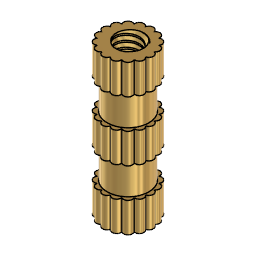
colour_detection_mechanism (Autodesk Fusion 360 archive; units mm, degrees)
design "M2 10 mm Threaded Brass Insert"
part number: 2026-06-20-09-24-02-047
Autodesk Fusion 360 part; units mm, degrees
sketch "Brass thread outline" plane through (0, 0, 0) normal (0, 0, 1) x (1, 0, 0)
  circle A0 centre (0, 0) radius 1.4
  dimension "d4" = 2.8
  constraint coincident A0.centre origin
  measures "d4" diameter of A0
extrude "Extrude1" add sketch "Brass thread outline" along normal blind 10
sketch "Ridges" plane through (0, 0, 10) normal (0, 0, 1) x (-1, 0, 0)
  circle A0 centre (0, 0) radius 1.4
  circle A1 centre (0, 0) radius 1.7
  circle A2 centre (-0.0001, -1.4) radius 0.3
  circle A3 centre (0.5357, -1.2935) radius 0.3
  circle A4 centre (0.9899, -0.99) radius 0.3
  circle A5 centre (1.2934, -0.5358) radius 0.3
  circle A6 centre (1.4, -0.0001) radius 0.3
  circle A7 centre (1.2935, 0.5357) radius 0.3
  circle A8 centre (0.99, 0.9899) radius 0.3
  circle A9 centre (0.5358, 1.2934) radius 0.3
  circle A10 centre (0.0001, 1.4) radius 0.3
  circle A11 centre (-0.5357, 1.2935) radius 0.3
  circle A12 centre (-0.9899, 0.99) radius 0.3
  circle A13 centre (-1.2934, 0.5358) radius 0.3
  circle A14 centre (-1.4, 0.0001) radius 0.3
  circle A15 centre (-1.2935, -0.5357) radius 0.3
  circle A16 centre (-0.99, -0.9899) radius 0.3
  circle A17 centre (-0.5358, -1.2934) radius 0.3
  dimension "d8" = 3.4
  dimension "d29" = 0.0001
  dimension "d31" = 360
  constraint coincident A0.centre A1.centre
  constraint coincident A0 A2.centre
  constraint tangent A1 A2
  measures "d8" diameter of A1
  measures "d29" horizontal distance of A0.centre A2.centre
extrude "Extrude2" add sketch "Ridges" against normal blind 2 contours A0 A5 A6 A7 | A0 A5 A6 A7 | A0 A6 A7 | A0 A6 A7 | A0 A5 A6 | A0 A5 A6 | A0 A6 A7 A8 | A0 A6 A7 A8 | A2 A3 A4 A5 A6 A7 A8 A9 A10 A11 A12 A13 A14 A15 A16 A17 | A0 A4 A5 A6 | A0 A4 A5 A6 | A0 A7 A8 | A0 A7 A8 | A0 A7 A8 A9 | A0 A4 A5 | A0 A4 A5 | A0 A3 A4 A5 | A0 A7 A8 A9 | A0 A8 A9 A10 | A0 A8 A9 | A0 A3 A4 A5 | A0 A2 A3 A4 | A0 A3 A4 | A0 A8 A9 | A0 A8 A9 A10 | A0 A9 A10 A11 | A0 A9 A10 | A0 A3 A4 | A0 A2 A3 A17 | A0 A2 A3 | A0 A2 A3 A4 | A0 A9 A10 | A0 A9 A10 A11 | A0 A10 A11 A12 | A0 A10 A11 | A0 A2 A3 | A0 A2 A17 | A0 A2 A16 A17 | A0 A2 A3 A17 | A0 A10 A11 | A0 A10 A11 A12 | A0 A11 A12 A13 | A0 A11 A12 | A0 A2 A16 A17 | A0 A2 A17 | A0 A15 A16 A17 | A0 A16 A17 | A0 A11 A12 | A0 A11 A12 A13 | A0 A16 A17 | A0 A15 A16 A17 | A0 A12 A13 | A0 A12 A13 | A0 A12 A13 A14 | A0 A14 A15 A16 | A0 A15 A16 | A0 A15 A16 | A0 A12 A13 A14 | A0 A14 A15 A16 | A0 A13 A14 | A0 A13 A14 | A0 A13 A14 A15 | A0 A13 A14 A15 | A0 A14 A15 | A0 A14 A15
pattern_linear "R-Pattern1" count 3 spacing 4 along (0, 0, -1) of "Extrude2"
sketch "Thread hole" plane through (0, 0, 10) normal (0, 0, 1) x (-1, 0, 0)
  circle A0 centre (0, 0) radius 1
  arc A1 (0.292, -1.4685) -> (0.8317, -1.2449) centre (0.5357, -1.2935) ccw
  arc A2 (0.8317, -1.2449) -> (1.2448, -0.8319) centre (0.9899, -0.99) ccw
  arc A3 (1.2448, -0.8319) -> (1.4684, -0.2922) centre (1.2934, -0.5358) ccw
  arc A4 (1.4684, -0.2922) -> (1.4685, 0.292) centre (1.4, -0.0001) ccw
  arc A5 (1.4685, 0.292) -> (1.2449, 0.8317) centre (1.2935, 0.5357) ccw
  arc A6 (1.2449, 0.8317) -> (0.8319, 1.2448) centre (0.99, 0.9899) ccw
  arc A7 (0.8319, 1.2448) -> (0.2922, 1.4684) centre (0.5358, 1.2934) ccw
  arc A8 (0.2922, 1.4684) -> (-0.292, 1.4685) centre (0.0001, 1.4) ccw
  arc A9 (-0.292, 1.4685) -> (-0.8317, 1.2449) centre (-0.5357, 1.2935) ccw
  arc A10 (-0.8317, 1.2449) -> (-1.2448, 0.8319) centre (-0.9899, 0.99) ccw
  arc A11 (-1.2448, 0.8319) -> (-1.4684, 0.2922) centre (-1.2934, 0.5358) ccw
  arc A12 (-1.4684, 0.2922) -> (-1.4685, -0.292) centre (-1.4, 0.0001) ccw
  arc A13 (-1.4685, -0.292) -> (-1.2449, -0.8317) centre (-1.2935, -0.5357) ccw
  arc A14 (-1.2449, -0.8317) -> (-0.8319, -1.2448) centre (-0.99, -0.9899) ccw
  arc A15 (-0.8319, -1.2448) -> (-0.2922, -1.4684) centre (-0.5358, -1.2934) ccw
  arc A16 (-0.2922, -1.4684) -> (0.292, -1.4685) centre (-0.0001, -1.4) ccw
  dimension "d11" = 2
  constraint coincident A0.centre origin
  measures "d11" diameter of A0
extrude "Extrude3" cut sketch "Thread hole" against normal blind 10 contours A0
thread "Thread1" "ISO Metric profile 2.0 M2x0.4 M2x0.4 6H" major diameter 2.074 minor diameter 1.623 pitch 0.4 angle 60 modelled right hand crest width 0.1065 on face at (-0.9988, 0.0498, 3.3333) crest through (-0.8115, 0, 9.9)
equation "outer_diameter = 2.8 mm" comment "The outer diameter of the non-ridged parts."
equation "hole_diameter = 2 mm" comment "The thread diameter of the brass insert. 2 mm for this M2 insert."
equation "height = 10 mm" comment "The height of the brass thread insert. 10 mm for this model."
equation "d4 = outer_diameter"
equation "d5 = height"
equation "ridge_diameter = 3.4 mm" comment "The outer diameter of the ridged parts."
equation "d8 = ridge_diameter"
equation "d9 = -ridge_height"
equation "d11 = hole_diameter"
equation "d12 = -height"
equation "number_of_ridges = 3" comment "The number of ridges to have along the outside."
equation "d23 = number_of_ridges"
equation "d25 = -ridge_pattern_length"
equation "ridge_pattern_length = height - ridge_height" comment "The distance to use for the rectangular pattern that repeats the ridges."
equation "ridge_height = 2 mm" comment "The height of the individual ridges."
named bodies: "M2 10 mm Threaded Brass Insert"

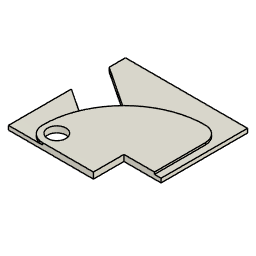
design "Colour Detection Mechanism Platform"
Autodesk Fusion 360 part; units mm, degrees
sketch "Colour Detection Mechanism Platform" plane through (0, 0, 0) normal (0, 0, 1) x (1, 0, 0)
  line L0 (0, 0) -> (120, 0)
  line L1 (120, 0) -> (120, 76)
  line L2 (120, 76) -> (0, 76)
  line L3 (0, 76) -> (0, 0)
  dimension "d169" = 120
  dimension "d170" = 76
  constraint horizontal L0
  constraint vertical L1
  constraint horizontal L2
  constraint vertical L3
  constraint coincident L0.start L3.end
  measures "d169" distance of L0.start L0.end
  measures "d170" distance of L0.start L2.end
extrude "Extrude42" add sketch "Colour Detection Mechanism Platform" along normal blind 4
sketch "Smartie Path" plane through (0, 0, 4) normal (0, 0, 1) x (-1, 0, 0)
  line L0 (0, -76) -> (0, 0)
  line L1 (0, 0) -> (-120, 0)
  line L2 (-120, 0) -> (-120, -76)
  line L3 (-120, -76) -> (0, -76)
  circle A0 centre (-98.5, 24) radius 80
  line L4 (-98.5, 24) -> (-113.5, 24)
  line L5 (-113.5, 24) -> (-113.5, -56)
  line L6 (-113.5, -56) -> (-98.5, -56)
  line L7 (-98.5, -56) -> (-98.5, 24)
  line L8 (-98.5, 24) -> (-18.5, 24)
  line L9 (-18.5, 24) -> (-18.5, 39)
  line L10 (-18.5, 39) -> (-98.5, 39)
  line L11 (-98.5, 39) -> (-98.5, 24)
  line L12 (-98.5, 24) -> (-113.5, 24)
  line L13 (-113.5, 24) -> (-113.5, 39)
  line L14 (-113.5, 39) -> (-98.5, 39)
  line L15 (-98.5, 39) -> (-98.5, 24)
  circle A1 centre (-32.5, 24) radius 9
  dimension "d173" = 160
  dimension "d174" = 24
  dimension "d175" = 21.5
  dimension "d176" = 15
  dimension "d177" = 15
  dimension "d178" = 80
  dimension "d179" = 80
  dimension "d184" = 18
  dimension "d185" = 14
  constraint horizontal L4
  constraint vertical L5
  constraint horizontal L6
  constraint vertical L7
  constraint coincident A0.centre L4.start
  constraint horizontal L8
  constraint vertical L9
  constraint horizontal L10
  constraint vertical L11
  constraint horizontal L12
  constraint vertical L13
  constraint horizontal L14
  constraint vertical L15
  constraint collinear L5 L13
  constraint collinear L10 L14
  constraint coincident L8 A1.centre
  measures "d173" diameter of A0
  measures "d174" distance of L1 A0.centre
  measures "d175" horizontal distance of L1.end A0.centre
  measures "d176" distance of L8.end L9.end
  measures "d177" distance of L5.end L6.end
  measures "d178" distance of L4.end L5.end
  measures "d179" distance of L9.end L10.end
  measures "d184" diameter of A1
  measures "d185" distance of L8.end A1.centre
extrude "Extrude43" add sketch "Smartie Path" along normal blind 2 contours L1 A0 L7 | L1 A0 L7 L8 A1 | L1 A0 L5 L7 | L1 L4 L5 L7 L12 | A0 L8 L10 L11 L15 A1 | L4 L11 L12 L13 L14 L15
fillet "Fillet2" radius 15 2 edges at (19.9188, -39, 5) (113.5, 54.5812, 5)
extrude "Extrude44" add 1 faces at (89.4665, -20.5529, 4) along direction (0, 0, -1) blind 4
sketch "Servo Hole" plane through (0, 0, 6) normal (0, 0, 1) x (-1, 0, 0)
  circle A0 centre (-32.5, 24) radius 9
  arc A1 (-113.5, -41) -> (-98.5, -56) centre (-98.5, -41) ccw
  arc A2 (-98.5, -56) -> (-18.5, 24) centre (-98.5, 24) ccw
  arc A3 (-18.5, 24) -> (-33.5, 39) centre (-33.5, 24) ccw
  line L0 (-33.5, 39) -> (-113.5, 39)
  line L1 (-113.5, 39) -> (-113.5, -41)
  line L2 (-113.5, 39) -> (-83.5, 39)
  line L3 (-83.5, 39) -> (-83.5, 9)
  line L4 (-83.5, 9) -> (-113.5, 9)
  line L5 (-113.5, 9) -> (-113.5, 39)
  dimension "d188" = 30
  dimension "d189" = 30
  constraint horizontal L2
  constraint vertical L3
  constraint horizontal L4
  constraint vertical L5
  constraint coincident L0.end L1.start
  measures "d188" distance of L3.end L4.end
  measures "d189" distance of L2.end L3.end
extrude "Extrude45" cut sketch "Servo Hole" against normal blind 6 contours L0 L1 L2 L3 L4 L5
sketch "Colour Sensor Holder Hole" plane through (0, 0, 4) normal (0, 0, 1) x (-1, 0, 0)
  line L0 (-120, 0) -> (-120, -76)
  line L1 (-120, -76) -> (0, -76)
  line L2 (0, -76) -> (0, 0)
  line L3 (-113.5, 0) -> (-120, 0)
  arc A0 (-98.5, -56) -> (-22.1849, 0) centre (-98.5, 24) ccw
  arc A1 (-113.5, -41) -> (-98.5, -56) centre (-98.5, -41) ccw
  line L4 (-113.5, -41) -> (-113.5, 0)
  line L5 (0, -59.401) -> (-38.732, -33.6675)
  line L6 (0, -23.4021) -> (-22.139, -8.693)
  line L7 (-38.732, -33.6675) -> (-22.139, -8.693)
  line L8 (0, -60.0013) -> (-39.4252, -33.8073)
  line L9 (-39.4252, -33.8073) -> (-22.2788, -7.9998)
  line L10 (-22.2788, -7.9998) -> (0, -22.8018)
  line L11 (0, 0) -> (-22.1849, 0)
  dimension "d249" = 56.4
  dimension "d250" = 59.401
  dimension "d254" = 56.4
  dimension "d255" = 8.693
  dimension "d256" = 22.139
  dimension "d257" = 23.4021
  dimension "d258" = 38.732
  dimension "d261" = 0.5
  dimension "d262" = 0.5
  dimension "d263" = 0.5
  constraint coincident L2 L5.start
  constraint coincident L2 L6.start
  constraint coincident L2 L8.start
  constraint coincident L2 L10.end
  constraint perpendicular L9 L10
  constraint parallel L5 L8
  constraint parallel L7 L9
  measures "d249" angle of L2 L5
  measures "d250" distance of L2.end L5.start
  measures "d254" angle of L2 L6
  measures "d255" distance of L3 L6.end
  measures "d256" horizontal distance of L2.end L6.end
  measures "d257" distance of L2.end L6.start
  measures "d258" horizontal distance of L5.start L5.end
  measures "d261" distance of L5 L8
  measures "d262" distance of L7 L9
extrude "Extrude58" cut sketch "Colour Sensor Holder Hole" against normal blind 4 contours L2 L5 L6 L7
extrude "Extrude59" cut sketch "Colour Sensor Holder Hole" against normal blind 4 contours L2 L5 L6 L7 L8 L9 L10
sketch "Platform Extension" plane through (0, 0, 4) normal (0, 0, 1) x (-1, 0, 0)
  line L0 (-22.2788, -7.9998) -> (0, -22.8018)
  line L1 (0, -22.8018) -> (0, 0)
  line L2 (0, 0) -> (-22.1849, 0)
  arc A0 (-98.5, -56) -> (-22.1849, 0) centre (-98.5, 24) ccw
  arc A1 (-113.5, -41) -> (-98.5, -56) centre (-98.5, -41) ccw
  line L3 (-113.5, -41) -> (-113.5, 0)
  line L4 (-120, 0) -> (-120, -76)
  line L5 (-120, -76) -> (0, -76)
  line L6 (0, -60.0013) -> (-39.4252, -33.8073)
  line L7 (-39.4252, -33.8073) -> (-22.2788, -7.9998)
  line L8 (-83.5, 9) -> (-113.5, 9)
  line L9 (-113.5, 9) -> (-113.5, -41)
  arc A2 (-113.5, -41) -> (-98.5, -56) centre (-98.5, -41) ccw
  arc A3 (-98.5, -56) -> (-18.5, 24) centre (-98.5, 24) ccw
  arc A4 (-18.5, 24) -> (-33.5, 39) centre (-33.5, 24) ccw
  line L10 (-33.5, 39) -> (-83.5, 39)
  line L11 (-83.5, 39) -> (-83.5, 9)
  circle A5 centre (-32.5, 24) radius 9
  line L12 (0, 0) -> (0, 39)
  line L13 (0, 39) -> (-33.5, 39)
  line L14 (-113.5, 0) -> (-120, 0)
  line L15 (0, -76) -> (0, -60.0013)
  line L16 (-113.5, 0) -> (-120, 0)
  line L17 (-120, 0) -> (-120, 9)
  line L18 (-120, 9) -> (-113.5, 9)
  line L19 (-113.5, 9) -> (-113.5, 0)
  constraint coincident L1.end L2.start
  constraint coincident A4.end L10.start
  constraint perpendicular L2 L12
  constraint perpendicular L12 L13
  constraint horizontal L16
  constraint vertical L17
  constraint horizontal L18
  constraint vertical L19
  constraint coincident L3.end L14.start
  constraint collinear L4 L17
  constraint collinear L8 L18
extrude "Extrude60" add sketch "Platform Extension" against normal blind 4 contours L2 A3 A4 L12 L13 | L9 L14 L16 L17 L18 L19
equation "d95 = 4 mm + 1.5 mm"
equation "d103 = -( 29 mm - 16 mm )"
named bodies: "Colour Detection Mechanism Platform"

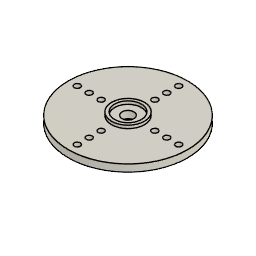
design "Savöx SH 0255 MG Micro Servo Horn"
description: Spur Gear; Module: 0.217; Num Teeth: 21; Pressure Angle: 20.0; Backlash: 0.00 mm
part number: 2026-07-12-11-53-48-100
Autodesk Fusion 360 part; units mm, degrees
sketch "Horn body" plane through (0, 0, 0) normal (0, 0, 1) x (1, 0, 0)
  circle A0 centre (0, 0) radius 10
  dimension "d1" = 20
  constraint coincident A0.centre origin
  measures "d1" diameter of A0
extrude "Extrude1" add sketch "Horn body" along normal blind 1.2 makes body 1
sketch "Connector" plane through (0, 0, 0) normal (0, 0, -1) x (1, 0, 0)
  circle A0 centre (0, 0) radius 10
  circle A1 centre (0, 0) radius 3.5
  dimension "d5" = 7
  constraint coincident A0.centre A1.centre
  measures "d5" diameter of A1
extrude "Extrude2" add sketch "Connector" along normal blind 3 contours A1 bodies 1
sketch "Screw hole" plane through (0, 0, 1.2) normal (0, 0, 1) x (-1, 0, 0)
  circle A0 centre (0, 0) radius 10
  circle A1 centre (0, 0) radius 2.75
  circle A2 centre (0, 0) radius 2.25
  circle A3 centre (0, 0) radius 1
  dimension "d8" = 5.5
  dimension "d9" = 4.5
  dimension "d10" = 2
  constraint coincident A0.centre A1.centre
  constraint concentric A2 A3
  measures "d8" diameter of A1
  measures "d9" diameter of A2
  measures "d10" diameter of A3
extrude "Extrude3" add sketch "Screw hole" along normal blind 0.5 contours A1 bodies 1
extrude "Extrude4" cut sketch "Screw hole" against normal blind 1.2 contours A3 bodies 1
sketch "Top small holes" plane through (0, 0, 1.2) normal (0, 0, 1) x (-1, 0, 0)
  circle A0 centre (0, 0) radius 10
  circle A1 centre (0, 0) radius 2.75
  circle A2 centre (0, -8.5) radius 0.5
  circle A3 centre (0, -6.5) radius 0.5
  circle A4 centre (0, -4.5) radius 0.5
  dimension "d15" = 1
  dimension "d16" = 1
  dimension "d17" = 1
  dimension "d19" = 8.5
  dimension "d20" = 6.5
  dimension "d21" = 4.5
  measures "d15" diameter of A2
  measures "d16" diameter of A3
  measures "d17" diameter of A4
  measures "d19" distance of A0.centre A2.centre
  measures "d20" distance of A0.centre A3.centre
  measures "d21" distance of A0.centre A4.centre
extrude "Extrude5" cut sketch "Top small holes" against normal blind 1.2 contours A2 | A3 | A4 bodies 1
pattern_circular "C-Pattern1" count 4 over 360 about axis through (0, 0, 1.75) along (0, 0, 1) of "Extrude5"
sketch "Base Circle" plane through (0, 0, 0) normal (0, 0, 1) x (1, 0, 0) in component "Savöx SH 0255 MG Micro Servo Gear"
  circle A0 centre (0, 0) radius 2.0274
extrude "Extrude1'" add sketch "Base Circle" along normal blind 3 separate body makes body 2 in component "Savöx SH 0255 MG Micro Servo Gear"
sketch "Gear Tooth" plane through (0, 0, 0) normal (0, 0, 1) x (1, 0, 0) in component "Savöx SH 0255 MG Micro Servo Gear"
  spline S0 degree 5 poles (2.1325, -0.1918) (2.1335, -0.1919) (2.1355, -0.1921) (2.1386, -0.1922) (2.1427, -0.1923) (2.1478, -0.1921) (2.1529, -0.1919) (2.1581, -0.1915) (2.1632, -0.191) (2.1683, -0.1906) (2.1735, -0.1901) (2.1787, -0.1895) (2.1838, -0.1889) (2.189, -0.1882) (2.1941, -0.1875) (2.1993, -0.1867) (2.2045, -0.1858) (2.2097, -0.1849) (2.2148, -0.1839) (2.22, -0.1829) (2.2252, -0.1818) (2.2304, -0.1807) (2.2356, -0.1796) (2.2407, -0.1784) (2.2459, -0.1772) (2.2511, -0.1759) (2.2563, -0.1746) (2.2615, -0.1732) (2.2667, -0.1718) (2.2719, -0.1703) (2.2771, -0.1689) (2.2823, -0.1674) (2.2875, -0.1658) (2.2927, -0.1642) (2.2979, -0.1626) (2.3031, -0.1609) (2.3083, -0.1592) (2.3134, -0.1575) (2.3186, -0.1557) (2.3238, -0.1539) (2.329, -0.152) (2.3342, -0.1502) (2.3394, -0.1482) (2.3446, -0.1463) (2.3498, -0.1443) (2.355, -0.1423) (2.3602, -0.1403) (2.3654, -0.1382) (2.3705, -0.1361) (2.3757, -0.1339) (2.3809, -0.1317) (2.3861, -0.1295) (2.3913, -0.1273) (2.3964, -0.125) (2.4016, -0.1227) (2.4068, -0.1204) (2.412, -0.118) (2.4171, -0.1156) (2.4223, -0.1132) (2.4275, -0.1107) (2.4326, -0.1082) (2.4378, -0.1057) (2.4429, -0.1032) (2.4481, -0.1006) (2.4532, -0.098) (2.4584, -0.0953) (2.4635, -0.0927) (2.4687, -0.09) (2.4738, -0.0872) (2.479, -0.0845) (2.4841, -0.0817) (2.4882, -0.0794) (2.4913, -0.0777) (2.4933, -0.0766) (2.4943, -0.076) knots 0 0 0 0 0 0 0.01428571 0.02857143 0.04285714 0.05714286 0.07142857 0.08571429 0.1 0.11428571 0.12857143 0.14285714 0.15714286 0.17142857 0.18571429 0.2 0.21428571 0.22857143 0.24285714 0.25714286 0.27142857 0.28571429 0.3 0.31428571 0.32857143 0.34285714 0.35714286 0.37142857 0.38571429 0.4 0.41428571 0.42857143 0.44285714 0.45714286 0.47142857 0.48571429 0.5 0.51428571 0.52857143 0.54285714 0.55714286 0.57142857 0.58571429 0.6 0.61428571 0.62857143 0.64285714 0.65714286 0.67142857 0.68571429 0.7 0.71428571 0.72857143 0.74285714 0.75714286 0.77142857 0.78571429 0.8 0.81428571 0.82857143 0.84285714 0.85714286 0.87142857 0.88571429 0.9 0.91428571 0.92857143 0.94285714 0.95714286 0.97142857 0.98571429 1 1 1 1 1 1
  spline S1 degree 5 poles (2.1325, 0.1918) (2.1335, 0.1919) (2.1355, 0.1921) (2.1386, 0.1922) (2.1427, 0.1923) (2.1478, 0.1921) (2.1529, 0.1919) (2.1581, 0.1915) (2.1632, 0.191) (2.1683, 0.1906) (2.1735, 0.1901) (2.1787, 0.1895) (2.1838, 0.1889) (2.189, 0.1882) (2.1941, 0.1875) (2.1993, 0.1867) (2.2045, 0.1858) (2.2097, 0.1849) (2.2148, 0.1839) (2.22, 0.1829) (2.2252, 0.1818) (2.2304, 0.1807) (2.2356, 0.1796) (2.2407, 0.1784) (2.2459, 0.1772) (2.2511, 0.1759) (2.2563, 0.1746) (2.2615, 0.1732) (2.2667, 0.1718) (2.2719, 0.1703) (2.2771, 0.1689) (2.2823, 0.1674) (2.2875, 0.1658) (2.2927, 0.1642) (2.2979, 0.1626) (2.3031, 0.1609) (2.3083, 0.1592) (2.3134, 0.1575) (2.3186, 0.1557) (2.3238, 0.1539) (2.329, 0.152) (2.3342, 0.1502) (2.3394, 0.1482) (2.3446, 0.1463) (2.3498, 0.1443) (2.355, 0.1423) (2.3602, 0.1403) (2.3654, 0.1382) (2.3705, 0.1361) (2.3757, 0.1339) (2.3809, 0.1317) (2.3861, 0.1295) (2.3913, 0.1273) (2.3964, 0.125) (2.4016, 0.1227) (2.4068, 0.1204) (2.412, 0.118) (2.4171, 0.1156) (2.4223, 0.1132) (2.4275, 0.1107) (2.4326, 0.1082) (2.4378, 0.1057) (2.4429, 0.1032) (2.4481, 0.1006) (2.4532, 0.098) (2.4584, 0.0953) (2.4635, 0.0927) (2.4687, 0.09) (2.4738, 0.0872) (2.479, 0.0845) (2.4841, 0.0817) (2.4882, 0.0794) (2.4913, 0.0777) (2.4933, 0.0766) (2.4943, 0.076) knots 0 0 0 0 0 0 0.01428571 0.02857143 0.04285714 0.05714286 0.07142857 0.08571429 0.1 0.11428571 0.12857143 0.14285714 0.15714286 0.17142857 0.18571429 0.2 0.21428571 0.22857143 0.24285714 0.25714286 0.27142857 0.28571429 0.3 0.31428571 0.32857143 0.34285714 0.35714286 0.37142857 0.38571429 0.4 0.41428571 0.42857143 0.44285714 0.45714286 0.47142857 0.48571429 0.5 0.51428571 0.52857143 0.54285714 0.55714286 0.57142857 0.58571429 0.6 0.61428571 0.62857143 0.64285714 0.65714286 0.67142857 0.68571429 0.7 0.71428571 0.72857143 0.74285714 0.75714286 0.77142857 0.78571429 0.8 0.81428571 0.82857143 0.84285714 0.85714286 0.87142857 0.88571429 0.9 0.91428571 0.92857143 0.94285714 0.95714286 0.97142857 0.98571429 1 1 1 1 1 1
  arc A0 (2.4943, -0.076) -> (2.4943, 0.076) centre (0, 0) ccw
  line L0 (2.0093, -0.1807) -> (2.1325, -0.1918)
  line L1 (2.0093, 0.1807) -> (2.1325, 0.1918)
  line L2 (2.0093, -0.1807) -> (2.0093, 0.1807)
  point P0 (2.1579, -0.1915)
  point P1 (2.1836, -0.1889)
  point P2 (2.2093, -0.1849)
  point P3 (2.2351, -0.1797)
  point P4 (2.261, -0.1733)
  point P5 (2.287, -0.1659)
  point P6 (2.3129, -0.1576)
  point P7 (2.3389, -0.1484)
  point P8 (2.3649, -0.1384)
  point P9 (2.3908, -0.1275)
  point P10 (2.4168, -0.1158)
  point P11 (2.4427, -0.1033)
  point P12 (2.4685, -0.09)
  point P13 (2.1579, 0.1915)
  point P14 (2.1836, 0.1889)
  point P15 (2.2093, 0.1849)
  point P16 (2.2351, 0.1797)
  point P17 (2.261, 0.1733)
  point P18 (2.287, 0.1659)
  point P19 (2.3129, 0.1576)
  point P20 (2.3389, 0.1484)
  point P21 (2.3649, 0.1384)
  point P22 (2.3908, 0.1275)
  point P23 (2.4168, 0.1158)
  point P24 (2.4427, 0.1033)
  point P25 (2.4685, 0.09)
extrude "Extrude2'" add sketch "Gear Tooth" along normal blind 3 bodies 2 in component "Savöx SH 0255 MG Micro Servo Gear"
fillet "Fillet1" radius 0.1 2 edges at (2.0193, -0.1816, 1.5) (2.0193, 0.1816, 1.5) on bodies 2 in component "Savöx SH 0255 MG Micro Servo Gear"
pattern_circular "C-Pattern1'" count 21 over 360 about axis through (0, 0, 0) along (0, 0, 1) of "Extrude2'", "Fillet1" in component "Savöx SH 0255 MG Micro Servo Gear"
sketch "Diametrial Pitch Circle" plane through (0, 0, 0) normal (0, 0, 1) x (1, 0, 0) in component "Savöx SH 0255 MG Micro Servo Gear"
  circle A0 centre (0, 0) radius 2.2785 construction
move_body "Move1" bodies 2 to x (1, 0, 0) y (0, 1, 0) z (0, 0, 1) at (0, 0, -3) in component "Savöx SH 0255 MG Micro Servo Gear"
combine "Combine1" operation cut target body 1 tool bodies 2 keep tools
component "Savöx SH 0255 MG Micro Servo Gear" placed x (1, 0, 0) y (0, 1, 0) z (0, 0, 1) at (0, 0, 0)
named bodies: "Savöx SH 0255 MG Micro Servo Horn", "Savöx SH 0255 MG Micro Servo Gear"

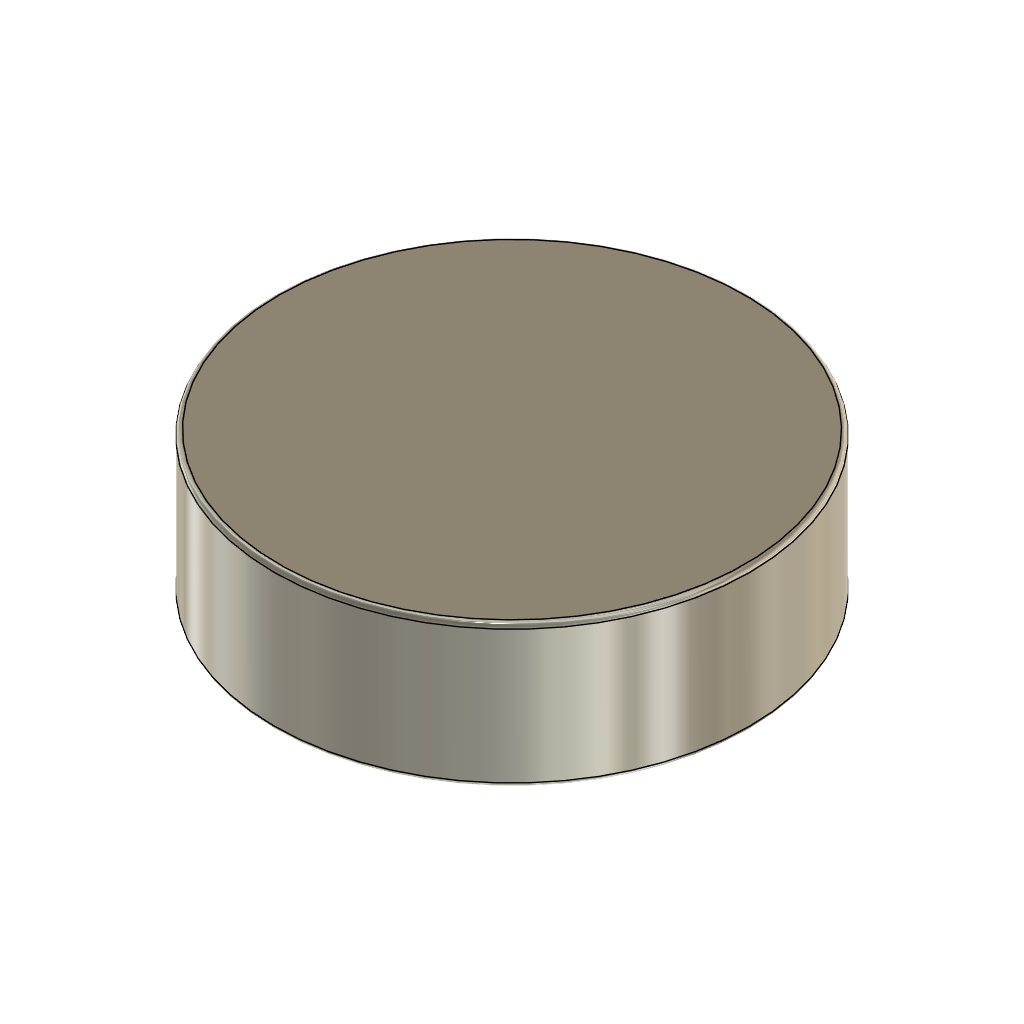
design "5 mm x 1.5 mm Neodymium Disc Magnet"
Autodesk Fusion 360 part; units mm, degrees
sketch "5 mm x 1.5 mm neodymium disc magnet" plane through (0, 0, 0) normal (0, 0, 1) x (1, 0, 0)
  circle A0 centre (0, 0) radius 2.5
  dimension "d1" = 5
  constraint coincident A0.centre origin
  measures "d1" diameter of A0
extrude "Extrude1" add sketch "5 mm x 1.5 mm neodymium disc magnet" along normal blind 1.5
fillet "Fillet1" radius 0.05 2 edges at (-2.3308, -0.904, 1.5) (-2.3308, -0.904, 0)
named bodies: "5 mm x 1.5 mm Neodymium Disc Magnet"
